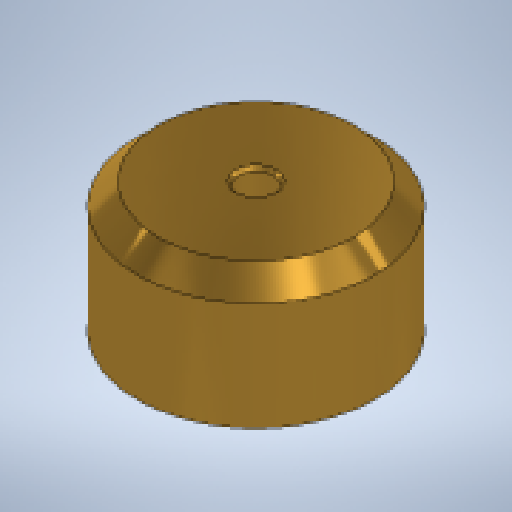
# Autodesk Inventor part: Flywheel
Saved by Autodesk Inventor 2023.4 (Build 274418000, 418)
## iProperties
Created: 2024-05-27
Part Number: Flywheel
Material: Brass, Soft Yellow
Document SubType Name: Modeling
Designer: Nathan Cai
Mass: 90.1087 g
Surface Area: 48.5291 cm^2
Volume: 10.6386 cm^3
Density: 8.47 g/cm^3
Appearance: Brass - Satin
Author: Nathan Cai
Autodesk Inventor part; units mm, degrees
ref_plane "YZ Plane" through (0, 0, 0) normal (1, 0, 0) x (0, 1, 0)
ref_plane "XZ Plane" through (0, 0, 0) normal (0, 1, 0) x (-1, 0, 0)
ref_plane "XY Plane" through (0, 0, 0) normal (0, 0, 1) x (1, 0, 0)
sketch "Sketch1" plane through (0, 0, 0) normal (0, 0, 1) x (1, 0, 0)
  line L0 (0, 0) -> (13.925, 0)
  line L1 (13.925, 0) -> (13.925, 11.5)
  line L2 (13.925, 11.5) -> (0, 11.5)
  line L3 (0, 11.5) -> (0, 0)
  line L4 (0, 0) -> (2.5, 0)
  line L5 (2.5, 0) -> (2.5, 25.4)
  line L6 (2.5, 25.4) -> (0, 25.4)
  line L7 (0, 25.4) -> (0, 0)
  line L8 (0, 0) -> (17.5, 0)
  line L9 (17.5, 0) -> (17.5, 19.05)
  line L10 (17.5, 19.05) -> (0, 19.05)
  line L11 (0, 19.05) -> (0, 0)
  line L12 (13.925, 11.5) -> (12.5, 11.5)
  line L13 (12.5, 11.5) -> (12.5, 7.5)
  line L14 (12.5, 7.5) -> (13.925, 7.5)
  line L15 (13.925, 7.5) -> (13.925, 11.5)
  point P0 (2.5, 19.05)
  point P1 (2.5, 11.5)
  point P2 (13.925, 0)
  dimension "d0" = 13.925
  dimension "d1" = 11.5
  dimension "d2" = 2.5
  dimension "d3" = 25.4
  dimension "d4" = 17.5
  dimension "d5" = 19.05
  dimension "d6" = 4
  dimension "d7" = 12.5
  constraints: 32 end point, 8 parallel, 4 horizontal, 4 perpendicular
  measures "d0" distance of L2.end L1.end
  measures "d1" distance of L1.end L0.end
  measures "d2" distance of L6.end L5.end
  measures "d3" distance of L5.end L4.end
  measures "d4" distance of L10.end L9.end
  measures "d5" distance of L9.end L8.end
  measures "d6" distance of L13.end L12.end
  measures "d7" distance between parallel lines of L7 L13
revolve "Revolution1" add sketch "Sketch1" angle 360 about axis through (0, 19.05, 0) along (0, -1, 0) contours L1 L2 L5 L10 L9 L8
chamfer "Chamfer1" distance 3.175 angle 45 1 edges at (-17.5, 19.05, 0)
chamfer "Chamfer2" distance 0.5 angle 45 3 edges at (-13.925, 0, 0) (-2.5, 11.5, 0) (-2.5, 19.05, 0)
body "Solid1"
